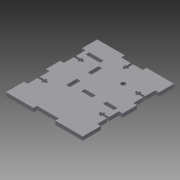
# Autodesk Inventor part: left
Saved by Autodesk Inventor 2014 (Build 180170000, 170)
## iProperties
Created: 2014-03-06
Part Number: left
Material: 常规
Document SubType Name: Modeling
Designer: Keshuai
Density: 1 g/cm^3
Appearance: 默认
Author: Keshuai
Autodesk Inventor part; units mm, degrees
ref_plane "YZ Plane" through (0, 0, 0) normal (1, 0, 0) x (0, 1, 0)
ref_plane "XZ Plane" through (0, 0, 0) normal (0, 1, 0) x (-1, 0, 0)
ref_plane "XY Plane" through (0, 0, 0) normal (0, 0, 1) x (1, 0, 0)
sketch "草图1" plane through (0, 0, 0) normal (0, 0, 1) x (1, 0, 0)
  circle A0 centre (37.7249, -83) radius 3.6 projected
  line L0 (65, -83) -> (65, -51) projected
  line L1 (65, -51) -> (47, -51) projected
  line L2 (47, -51) -> (47, -83) projected
  line L3 (47, -83) -> (65, -83) projected
  line L4 (89.2, -11.5) -> (96, -11.5) projected
  line L5 (96, -25) -> (96, -11.5) projected
  line L6 (96, -25) -> (101, -25) projected
  line L7 (101, -25) -> (101, -45) projected
  line L8 (96, -45) -> (101, -45) projected
  line L9 (96, -58.5) -> (96, -45) projected
  line L10 (96, -58.5) -> (89.2, -58.5) projected
  line L11 (89.2, -58.5) -> (89.2, -56.75) projected
  line L12 (89.2, -56.75) -> (86.8, -56.75) projected
  line L13 (86.8, -56.75) -> (86.8, -58.5) projected
  line L14 (86.8, -58.5) -> (84, -58.5) projected
  line L15 (84, -58.5) -> (84, -61.5) projected
  line L16 (84, -61.5) -> (86.8, -61.5) projected
  line L17 (86.8, -61.5) -> (86.8, -63.25) projected
  line L18 (86.8, -63.25) -> (89.2, -63.25) projected
  line L19 (89.2, -63.25) -> (89.2, -61.5) projected
  line L20 (89.2, -61.5) -> (96, -61.5) projected
  line L21 (96, -75) -> (96, -61.5) projected
  line L22 (96, -75) -> (101, -75) projected
  line L23 (101, -75) -> (101, -100) projected
  line L24 (101, -100) -> (63, -100) projected
  line L25 (63, -95) -> (63, -100) projected
  line L26 (33, -95) -> (63, -95) projected
  line L27 (33, -95) -> (33, -100) projected
  line L28 (33, -100) -> (-5, -100) projected
  line L29 (-5, -75) -> (-5, -100) projected
  line L30 (0, -75) -> (-5, -75) projected
  line L31 (0, -75) -> (0, -61.5) projected
  line L32 (0, -61.5) -> (6.8, -61.5) projected
  line L33 (6.8, -61.5) -> (6.8, -63.25) projected
  line L34 (6.8, -63.25) -> (9.2, -63.25) projected
  line L35 (9.2, -63.25) -> (9.2, -61.5) projected
  line L36 (9.2, -61.5) -> (12, -61.5) projected
  line L37 (12, -61.5) -> (12, -58.5) projected
  line L38 (12, -58.5) -> (9.2, -58.5) projected
  line L39 (9.2, -58.5) -> (9.2, -56.75) projected
  line L40 (9.2, -56.75) -> (6.8, -56.75) projected
  line L41 (6.8, -56.75) -> (6.8, -58.5) projected
  line L42 (6.8, -58.5) -> (0, -58.5) projected
  line L43 (0, -58.5) -> (0, -45) projected
  line L44 (0, -45) -> (-5, -45) projected
  line L45 (-5, -45) -> (-5, -25) projected
  line L46 (0, -25) -> (-5, -25) projected
  line L47 (0, -25) -> (0, -11.5) projected
  line L48 (0, -11.5) -> (6.8, -11.5) projected
  line L49 (6.8, -11.5) -> (6.8, -13.25) projected
  line L50 (6.8, -13.25) -> (9.2, -13.25) projected
  line L51 (9.2, -13.25) -> (9.2, -11.5) projected
  line L52 (9.2, -11.5) -> (12, -11.5) projected
  line L53 (12, -11.5) -> (12, -8.5) projected
  line L54 (12, -8.5) -> (9.2, -8.5) projected
  line L55 (9.2, -8.5) -> (9.2, -6.75) projected
  line L56 (9.2, -6.75) -> (6.8, -6.75) projected
  line L57 (6.8, -6.75) -> (6.8, -8.5) projected
  line L58 (6.8, -8.5) -> (0, -8.5) projected
  line L59 (0, -8.5) -> (0, 5) projected
  line L60 (0, 5) -> (-5, 5) projected
  line L61 (-5, 5) -> (-5, 26) projected
  line L62 (33, 26) -> (-5, 26) projected
  line L63 (33, 21) -> (33, 26) projected
  line L64 (33, 21) -> (46.5, 21) projected
  line L65 (46.5, 21) -> (46.5, 14.2) projected
  line L66 (46.5, 14.2) -> (44.75, 14.2) projected
  line L67 (44.75, 14.2) -> (44.75, 11.8) projected
  line L68 (44.75, 11.8) -> (46.5, 11.8) projected
  line L69 (46.5, 11.8) -> (46.5, 9) projected
  line L70 (46.5, 9) -> (49.5, 9) projected
  line L71 (49.5, 9) -> (49.5, 11.8) projected
  line L72 (49.5, 11.8) -> (51.25, 11.8) projected
  line L73 (51.25, 11.8) -> (51.25, 14.2) projected
  line L74 (51.25, 14.2) -> (49.5, 14.2) projected
  line L75 (49.5, 14.2) -> (49.5, 21) projected
  line L76 (49.5, 21) -> (63, 21) projected
  line L77 (63, 21) -> (63, 26) projected
  line L78 (63, 26) -> (101, 26) projected
  line L79 (101, 26) -> (101, 5) projected
  line L80 (96, 5) -> (101, 5) projected
  line L81 (96, -8.5) -> (96, 5) projected
  line L82 (96, -8.5) -> (89.2, -8.5) projected
  line L83 (89.2, -8.5) -> (89.2, -6.75) projected
  line L84 (89.2, -6.75) -> (86.8, -6.75) projected
  line L85 (86.8, -6.75) -> (86.8, -8.5) projected
  line L86 (86.8, -8.5) -> (84, -8.5) projected
  line L87 (84, -8.5) -> (84, -11.5) projected
  line L88 (84, -11.5) -> (86.8, -11.5) projected
  line L89 (86.8, -11.5) -> (86.8, -13.25) projected
  line L90 (86.8, -13.25) -> (89.2, -13.25) projected
  line L91 (89.2, -13.25) -> (89.2, -11.5) projected
  line L92 (25, 0) -> (25, 5) projected
  line L93 (25, 5) -> (5, 5) projected
  line L94 (5, 5) -> (5, 0) projected
  line L95 (5, 0) -> (25, 0) projected
  line L96 (28, -35) -> (28, -50) projected
  line L97 (28, -50) -> (33, -50) projected
  line L98 (33, -50) -> (33, -35) projected
  line L99 (33, -35) -> (28, -35) projected
  line L100 (28, -5) -> (28, -20) projected
  line L101 (28, -20) -> (33, -20) projected
  line L102 (33, -20) -> (33, -5) projected
  line L103 (33, -5) -> (28, -5) projected
  line L104 (46, -42) -> (46, -47) projected
  line L105 (46, -47) -> (61, -47) projected
  line L106 (61, -47) -> (61, -42) projected
  line L107 (61, -42) -> (46, -42) projected
  line L108 (76, -42) -> (76, -47) projected
  line L109 (76, -47) -> (91, -47) projected
  line L110 (91, -47) -> (91, -42) projected
  line L111 (91, -42) -> (76, -42) projected
  circle A1 centre (66, -9) radius 3 projected
  point P0 (0, 0)
extrude "拉伸1" add sketch "草图1" along normal blind 5 contours A0 | L3 L2 L1 L0 | L4 L5 L6 L7 L8 L9 L10 L11 L12 L13 L14 L15 L16 L17 L18 L19 L20 L21 L22 L23 L24 L25 L26 L27 L28 L29 L30 L31 L32 L33 L34 L35 L36 L37 L38 L39 L40 L41 L42 L43 L44 L45 L46 L47 L48 L49 L50 L51 L52 L53 L54 L55 L56 L57 L58 L59 L60 L61 L62 L63 L64 L65 L66 L67 L68 L69 L70 L71 L72 L73 L74 L75 L76 L77 L78 L79 L80 L81 L82 L83 L84 L85 L86 L87 L88 L89 L90 L91
sketch "草图2" plane through (0, 0, 5) normal (0, 0, 1) x (1, 0, 0)
  circle A0 centre (66, -9) radius 3 projected
  line L0 (96, -25) -> (96, -11.5) projected
  circle A1 centre (55.0452, -9) radius 6
  line L1 (60.2413, -12) -> (66, -12)
  line L2 (60.2413, -6) -> (66, -6)
  point P0 (0, 0)
  dimension "d2" = 12
  constraints: 4 end point, 4 point on circle, 1 centre point, 1 parallel, 1 perpendicular
  measures "d2" diameter of A1
extrude "拉伸2" cut sketch "草图2" against normal through all contours A0 L1 A1 L2 | A1
